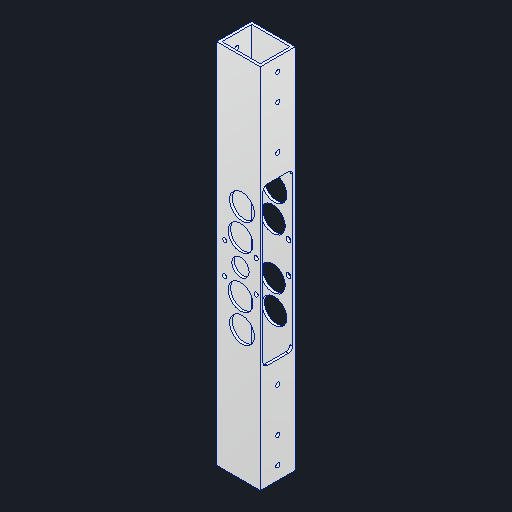
# Autodesk Inventor part: Wasp Mount Bar
Saved by Autodesk Inventor 2022 (Build 260153000, 153)
## iProperties
Created: 2022-09-18
Part Number: Wasp Mount Bar
Material: Generic
Document SubType Name: Modeling
Designer: robpl
Density: 1 g/cm^3
Appearance: Aluminum - Flat
Author: robpl
Autodesk Inventor part; units mm, degrees
ref_plane "YZ Plane" through (0, 0, 0) normal (1, 0, 0) x (0, 1, 0)
ref_plane "XZ Plane" through (0, 0, 0) normal (0, 1, 0) x (-1, 0, 0)
ref_plane "XY Plane" through (0, 0, 0) normal (0, 0, 1) x (1, 0, 0)
sketch "Sketch1" plane through (0, 0, 0) normal (0, 1, 0) x (-1, 0, 0)
  line L0 (0, 0) -> (50, 0)
  line L1 (50, 0) -> (50, -40)
  line L2 (50, -40) -> (0, -40)
  line L3 (0, -40) -> (0, 0)
  line L4 (3, -37) -> (47, -37)
  line L5 (47, -37) -> (47, -3)
  line L6 (47, -3) -> (3, -3)
  line L7 (3, -3) -> (3, -37)
  dimension "d0" = 50
  dimension "d1" = 40
  dimension "d2" = 3
  constraints: 16 end point, 4 parallel, 2 perpendicular, 1 horizontal, 3 other
  measures "d0" distance of L1.end L2.end
  measures "d1" distance of L0.end L1.end
  measures "d2" distance between parallel lines of L2 L4
extrude "Extrusion1" add sketch "Sketch1" along normal blind 420
sketch "Sketch2" plane through (0, 0, 0) normal (1, 0, 0) x (0, 0, -1)
  line L0 (0, 0) -> (40, 0) projected
  line L1 (40, 0) -> (40, 420) projected
  line L2 (0, 420) -> (40, 420) projected
  line L3 (0, 0) -> (0, 420) projected
  line L4 (3, 0) -> (3, 420) projected
  line L5 (37, 0) -> (37, 420) projected
  line L6 (3, 300) -> (37, 300)
  line L7 (37, 300) -> (37, 120)
  line L8 (37, 120) -> (3, 120)
  line L9 (3, 120) -> (3, 300)
  point P0 (3, 120)
  point P1 (37, 300)
  dimension "d5" = 120
  dimension "d6" = 120
  constraints: 8 end point, 2 parallel, 2 point on line, 1 horizontal, 1 perpendicular
  measures "d5" distance between parallel lines of L0 L8
  measures "d6" distance between parallel lines of L2 L6
extrude "Extrusion2" cut sketch "Sketch2" against normal blind 5 contours L4 L6 L5 L8
sketch "Sketch3" plane through (-50, 0, 0) normal (0, 0, 1) x (1, 0, 0)
  line L0 (0, 0) -> (50, 0) projected
  point P0 (27.2, 210)
  dimension "d9" = 210
  dimension "d10" = 27.2
  measures "d9" distance from line of L0 point (27.2, 210)
  measures "d10" horizontal distance of L0.start point (27.2, 210)
hole "Hole1" at (-22.8, 210, 0) direction (0, 0, -1) diameter 19 depth 8 tip angle 118 counterbore diameter 20 counterbore depth 5
sketch "Sketch4" plane through (-50, 0, -3) normal (0, 0, 1) x (1, 0, 0)
  circle A0 centre (27.2, 210) radius 10 projected
  circle A1 centre (27.2, 210) radius 25.4
  line L0 (8.6236, 227.3228) -> (44.5228, 228.5764)
  line L1 (44.5228, 228.5764) -> (45.7764, 192.6772)
  line L2 (45.7764, 192.6772) -> (9.8772, 191.4236)
  line L3 (9.8772, 191.4236) -> (8.6236, 227.3228)
  line L4 (8.6236, 227.3228) -> (45.7764, 192.6772) construction
  line L5 (44.5228, 228.5764) -> (9.8772, 191.4236) construction
  line L6 (50, 0) -> (50, 420) projected
  circle A2 centre (8.6236, 227.3228) radius 5.334
  circle A3 centre (44.5228, 228.5764) radius 5.334
  dimension "d18" = 50.8
  dimension "d19" = 2
  dimension "d34" = 10.668
  dimension "d35" = 10.668
  constraints: 12 end point, 5 coincident, 2 centre point, 2 midpoint, 2 parallel, 2 perpendicular, 3 other
  measures "d19" angle of L6 L1
  measures "d34" diameter of A2
  measures "d35" diameter of A3
hole "Hole2" [suppressed]
sketch "Sketch6" plane through (-3, 0, -3) normal (0, 0, -1) x (-1, 0, 0)
  circle A0 centre (37.1228, 191.4236) radius 5.334 projected
  circle A1 centre (38.3764, 227.3228) radius 5.334 projected
  circle A2 centre (2.4772, 228.5764) radius 5.334 projected
  point P0 (-3, 0)
  constraints: 3 coincident
hole "Hole4" [suppressed]
sketch "Sketch7" plane through (0, 0, -40) normal (0, 0, -1) x (-1, 0, 0)
  circle A0 centre (22.8, 210) radius 10 projected
  point P0 (0, 0)
  point P1 (22.8, 239.26)
  point P2 (22.8, 180.74)
  point P3 (21, 148.99)
  point P4 (21, 271.01)
  dimension "d45" = 31.75
  dimension "d46" = 1.8
  dimension "d47" = 31.75
  dimension "d94" = 29.26
  dimension "d95" = 29.26
  constraints: 3 vertical alignment
  measures "d45" vertical distance of point (22.8, 180.74) point (21, 148.99)
  measures "d46" horizontal distance of point (21, 148.99) point (22.8, 180.74)
  measures "d47" vertical distance of point (22.8, 239.26) point (21, 271.01)
  measures "d94" distance of point (22.8, 239.26) point (22.8, 210)
  measures "d95" distance of point (22.8, 180.74) point (22.8, 210)
hole "Hole5" at (-22.8, 239.26, -40) at (-22.8, 180.74, -40) at (-21, 148.99, -40) at (-21, 271.01, -40) direction (0, 0, 1) diameter 28.575 end through all
sketch "Sketch8" plane through (-3, 0, -3) normal (0, 0, -1) x (-1, 0, 0)
  circle A0 centre (19.8, 210) radius 25.4 construction
  line L0 (19.8, 210) -> (37.7605, 192.0395) construction
  line L1 (19.8, 210) -> (45.2, 210) construction
  circle A1 centre (19.8, 210) radius 10 projected
  point P0 (-3, 0)
  point P1 (37.7605, 227.9605)
  point P2 (1.8395, 227.9605)
  point P3 (1.8395, 192.0395)
  dimension "d55" = 50.8
  dimension "d56" = 45
  dimension "d59" = 360
  constraints: 4 end point, 3 coincident, 1 equal length, 1 horizontal, 8 other
  measures "d56" angle of L0 L1
hole "Hole6" at (-40.7605, 192.0395, -3) at (-40.7605, 227.9605, -3) at (-4.8395, 227.9605, -3) at (-4.8395, 192.0395, -3) direction (0, 0, 1) diameter 5 end through all
sketch "Sketch9" plane through (0, 0, -40) normal (0, 0, -1) x (-1, 0, 0)
  circle A0 centre (40.7605, 227.9605) radius 2.5 projected
  circle A1 centre (40.7605, 192.0395) radius 2.5 projected
  circle A2 centre (4.8395, 227.9605) radius 2.5 projected
  circle A3 centre (4.8395, 192.0395) radius 2.5 projected
  point P0 (0, 0)
  point P1 (40.7605, 192.0395)
  point P2 (4.8395, 192.0395)
  point P3 (4.8395, 227.9605)
  constraints: 4 coincident
hole "Hole7" at (-40.7605, 227.9605, -40) at (-40.7605, 192.0395, -40) at (-4.8395, 192.0395, -40) at (-4.8395, 227.9605, -40) direction (0, 0, 1) diameter 6 depth 8 tip angle 118
fillet "Fillet1" radius 5 4 edges at (-1.5, 300, -37) (-1.5, 300, -3) (-1.5, 120, -37) (-1.5, 120, -3)
sketch "Sketch11" plane through (-50, 0, -40) normal (-1, 0, 0) x (0, 0, 1)
  circle A0 centre (20, 95) radius 2.5 projected
  circle A1 centre (20, 375) radius 2.5 projected
  circle A2 centre (20, 45) radius 2.5 projected
  circle A3 centre (20, 15) radius 2.5 projected
  circle A4 centre (20, 405) radius 2.5 projected
  circle A5 centre (20, 325) radius 2.5 projected
  arc A6 (-45, 37) -> (-40, 32) centre (-40, 37) ccw projected
  line L0 (-40, 32) -> (-25, 32) projected
  arc A7 (-20, 27) -> (-25, 32) centre (-25, 27) ccw projected
  line L1 (-20, 27) -> (-20, -3) projected
  line L2 (10, -3) -> (-20, -3) projected
  arc A8 (15, -8) -> (10, -3) centre (10, -8) ccw projected
  line L3 (15, -40) -> (15, -8) projected
  line L4 (145, -40) -> (15, -40) projected
  line L5 (145, 460) -> (145, -40) projected
  line L6 (15, 460) -> (145, 460) projected
  line L7 (15, 428) -> (15, 460) projected
  arc A9 (10, 423) -> (15, 428) centre (10, 428) ccw projected
  line L8 (-15, 423) -> (10, 423) projected
  arc A10 (-15, 423) -> (-20, 418) centre (-15, 418) ccw projected
  line L9 (-20, 418) -> (-20, 393) projected
  arc A11 (-25, 388) -> (-20, 393) centre (-25, 393) ccw projected
  line L10 (-25, 388) -> (-40, 388) projected
  arc A12 (-40, 388) -> (-45, 383) centre (-40, 383) ccw projected
  line L11 (-45, 383) -> (-45, 318) projected
  arc A13 (-50, 313) -> (-45, 318) centre (-50, 318) ccw projected
  line L12 (-50, 313) -> (-113, 313) projected
  arc A14 (-118, 318) -> (-113, 313) centre (-113, 318) ccw projected
  line L13 (-118, 318) -> (-118, 418) projected
  arc A15 (-118, 418) -> (-123, 423) centre (-123, 418) ccw projected
  line L14 (-630, 423) -> (-123, 423) projected
  arc A16 (-635, 428) -> (-630, 423) centre (-630, 428) ccw projected
  line L15 (-635, 460) -> (-635, 428) projected
  line L16 (-755, 460) -> (-635, 460) projected
  line L17 (-755, -40) -> (-755, 460) projected
  line L18 (-635, -40) -> (-755, -40) projected
  line L19 (-635, -8) -> (-635, -40) projected
  arc A17 (-630, -3) -> (-635, -8) centre (-630, -8) ccw projected
  line L20 (-118, -3) -> (-630, -3) projected
  line L21 (-118, -3) -> (-118, 102) projected
  arc A18 (-113, 107) -> (-118, 102) centre (-113, 102) ccw projected
  line L22 (-113, 107) -> (-50, 107) projected
  arc A19 (-45, 102) -> (-50, 107) centre (-50, 102) ccw projected
  line L23 (-45, 102) -> (-45, 37) projected
  circle A20 centre (68.5, 440) radius 3 projected
  circle A21 centre (68.5, -20) radius 3 projected
  circle A22 centre (-742.5, 410) radius 2.5 projected
  circle A23 centre (-742.5, 210) radius 2.5 projected
  circle A24 centre (-742.5, 10) radius 2.5 projected
  circle A25 centre (132.5, 310) radius 2.5 projected
  circle A26 centre (132.5, 110) radius 2.5 projected
  circle A27 centre (-305, 12.5) radius 2.5 projected
  circle A28 centre (-485, 12.5) radius 2.5 projected
  circle A29 centre (-485, 407.5) radius 2.5 projected
  circle A30 centre (-305, 407.5) radius 2.5 projected
  circle A31 centre (-125, 407.5) radius 2.5 projected
  circle A32 centre (-125, 12.5) radius 2.5 projected
  circle A33 centre (132.5, 10) radius 2.5 projected
  circle A34 centre (132.5, 210) radius 2.5 projected
  circle A35 centre (132.5, 410) radius 2.5 projected
  circle A36 centre (-742.5, 110) radius 2.5 projected
  circle A37 centre (-742.5, 310) radius 2.5 projected
  circle A38 centre (33.5, -20) radius 3 projected
  circle A39 centre (33.5, 440) radius 3 projected
  arc A40 (40, 115) -> (35, 120) centre (35, 115) ccw projected
  line L24 (8, 120) -> (35, 120) projected
  arc A41 (3, 125) -> (8, 120) centre (8, 125) ccw projected
  line L25 (3, 295) -> (3, 125) projected
  arc A42 (8, 300) -> (3, 295) centre (8, 295) ccw projected
  line L26 (35, 300) -> (8, 300) projected
  arc A43 (35, 300) -> (40, 305) centre (35, 305) ccw projected
  line L27 (40, 393.2461) -> (40, 305) projected
  arc A44 (41.0957, 396.3696) -> (40, 393.2461) centre (45, 393.2461) ccw projected
  line L28 (58.4988, 418.1235) -> (41.0957, 396.3696) projected
  arc A45 (62.4031, 420) -> (58.4988, 418.1235) centre (62.4031, 415) ccw projected
  line L29 (115, 420) -> (62.4031, 420) projected
  arc A46 (120, 415) -> (115, 420) centre (115, 415) ccw projected
  line L30 (120, 5) -> (120, 415) projected
  arc A47 (115, 0) -> (120, 5) centre (115, 5) ccw projected
  line L31 (62.4031, 0) -> (115, 0) projected
  arc A48 (58.4988, 1.8765) -> (62.4031, 0) centre (62.4031, 5) ccw projected
  line L32 (41.0957, 23.6304) -> (58.4988, 1.8765) projected
  arc A49 (40, 26.7539) -> (41.0957, 23.6304) centre (45, 26.7539) ccw projected
  line L33 (40, 115) -> (40, 26.7539) projected
  point P0 (40, 0)
  point P1 (20, 405)
  point P2 (20, 375)
  point P3 (20, 325)
  point P4 (20, 95)
  point P5 (20, 45)
  point P6 (20, 15)
  constraints: 6 coincident
hole "Hole8" at (-50, 405, -20) at (-50, 375, -20) at (-50, 325, -20) at (-50, 95, -20) at (-50, 45, -20) at (-50, 15, -20) direction (1, 0, 0) diameter 5 end through all
equation "\"d6\" = d5"
equation "\"d47\" = d45"
equation "\"d95\" = d94"
body "Solid1"
